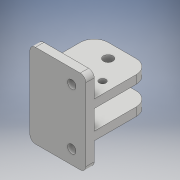
# Autodesk Inventor part: Część3
Saved by Autodesk Inventor 2017 (Build 210142000, 142)
## iProperties
Created: 2019-10-20
Part Number: Część3
Material: Ogólny
Document SubType Name: Modeling
Designer: patry
Density: 1 g/cm^3
Appearance: Domyślna
Author: patry
Autodesk Inventor part; units mm, degrees
ref_plane "YZ Plane" through (0, 0, 0) normal (1, 0, 0) x (0, 1, 0)
ref_plane "XZ Plane" through (0, 0, 0) normal (0, 1, 0) x (-1, 0, 0)
ref_plane "XY Plane" through (0, 0, 0) normal (0, 0, 1) x (1, 0, 0)
sketch "Szkic1" plane through (0, 0, 0) normal (0, 1, 0) x (-1, 0, 0)
  line L0 (15, 15) -> (-5, 15)
  line L1 (-5, 15) -> (-5, -15)
  line L2 (-5, -15) -> (15, -15)
  line L3 (15, -15) -> (15, 15)
  point P0 (0, 0)
  point P1 (0, 10)
  point P2 (0, -10)
  dimension "d0" = 20
  dimension "d1" = 20
  dimension "d2" = 15
  dimension "d3" = 5
  dimension "d4" = 5
  constraints: 8 end point, 2 parallel, 1 horizontal, 1 perpendicular, 1 vertical alignment, 1 other
  measures "d0" distance of point (0, -10) point (0, 10)
  measures "d1" distance of L1.end L2.end
  measures "d2" distance from line of L3 point (0, -10)
  measures "d3" distance from line of L0 point (0, 10)
  measures "d4" distance from line of L2 point (0, -10)
extrude "Wyciągnięcie proste1" add sketch "Szkic1" along normal blind 3
hole "Otwór1" at (0, 0, 10) at (0, 0, -10) direction (0, 1, 0) diameter 3 end through all
sketch "Szkic2" plane through (0, 3, 0) normal (0, 1, 0) x (1, 0, 0)
  circle A0 centre (0, -10) radius 1.5 projected
  circle A1 centre (0, 10) radius 1.5 projected
  line L0 (-15, -15) -> (5, -15) projected
  line L1 (5, -15) -> (5, 15) projected
  line L2 (5, 15) -> (-15, 15) projected
  line L3 (-15, 15) -> (-15, -15) projected
  line L4 (5, -15) -> (5, 15) projected
  line L5 (-15, -6.5) -> (5, -6.5)
  line L6 (5, -6.5) -> (5, -3.5)
  line L7 (5, -3.5) -> (-15, -3.5)
  line L8 (-15, -3.5) -> (-15, -6.5)
  line L9 (-15, 15) -> (-15, -15) projected
  line L10 (-15, 6.5) -> (5, 6.5)
  line L11 (5, 6.5) -> (5, 3.5)
  line L12 (5, 3.5) -> (-15, 3.5)
  line L13 (-15, 3.5) -> (-15, 6.5)
  point P0 (0, 0)
  dimension "d14" = 3
  dimension "d15" = 3
  dimension "d16" = 2
  dimension "d17" = 2
  constraints: 16 end point, 4 parallel, 4 point on line, 2 horizontal, 2 perpendicular
  measures "d14" distance between parallel lines of L10 L12
  measures "d15" distance between parallel lines of L7 L5
  measures "d16" distance edge to line of A0 L5
  measures "d17" distance edge to line of A1 L10
fillet "Zaokrąglenie1" radius 2 4 edges at (5, 1.5, 15) (-15, 1.5, 15) (5, 1.5, -15) (-15, 1.5, -15)
extrude "Wyciągnięcie proste2" add sketch "Szkic2" along normal blind 20 contours L3 L7 L1 L5 | L3 L10 L1 L12
fillet "Zaokrąglenie2" radius 5 4 edges at (-15, 23, 5) (5, 23, 5) (5, 23, -5) (-15, 23, -5)
sketch "Szkic3" plane through (-15, 3, 6.5) normal (0, 0, 1) x (1, 0, 0)
  arc A0 (5, 20) -> (0, 15) centre (5, 15) ccw projected
  line L0 (0, 0) -> (0, 15) projected
  line L1 (20, 0) -> (0, 0) projected
  line L2 (20, 0) -> (20, 15) projected
  arc A1 (20, 15) -> (15, 20) centre (15, 15) ccw projected
  line L3 (5, 20) -> (15, 20) projected
  point P0 (15, -3)
  point P1 (10, 15)
  dimension "d52" = 10
  measures "d52" distance from line of L0 point (10, 15)
hole "Otwór2" at (-5, 18, 6.5) direction (0, 0, -1) diameter 3.4 end through all clearance for "Śruba ze łbem płaskim obrobiona" size "M3" standard "ANSI Profil metryczny M"
sketch "Szkic4" plane through (-15, 3, 6.5) normal (0, 0, 1) x (1, 0, 0)
  arc A0 (5, 20) -> (0, 15) centre (5, 15) ccw projected
  line L0 (0, 0) -> (0, 15) projected
  line L1 (20, 0) -> (0, 0) projected
  line L2 (20, 0) -> (20, 15) projected
  circle A1 centre (10, 15.0001) radius 10 construction
  arc A2 (20, 15) -> (15, 20) centre (15, 15) ccw projected
  line L3 (5, 20) -> (15, 20) projected
  point P0 (15, -3)
  point P1 (6.0718, 5.804)
  point P2 (16, 7.0001)
  point P3 (11.1962, 5.0719)
  dimension "d33" = 20
  dimension "d53" = 30
  dimension "d54" = 30
  dimension "d62" = 4
  constraints: 3 point on circle, 1 centre point, 1 other
  measures "d33" diameter of A1
  measures "d62" distance from line of L2 point (16, 7)
hole "Otwór5" at (-8.9282, 8.804, 6.5) at (1, 10.0001, 6.5) at (-3.8038, 8.0719, 6.5) direction (0, 0, -1) diameter 2.4 end up to face face through (-5.0683, 7.4375, 3.5) facing (0, 0, -1) clearance for "Śruba ze łbem płaskim obrobiona" size "M2" standard "ANSI Profil metryczny M"
equation "\"d4\" = d3"
equation "\"d15\" = d14"
equation "\"d54\" = d53"
